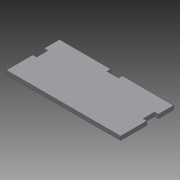
# Autodesk Inventor part: Controller_Top
Saved by Autodesk Inventor 2014 (Build 180170000, 170)
## iProperties
Created: 2014-11-10
Part Number: Controller_Top
Material: Generic
Document SubType Name: Modeling
Designer: ThatOtherGuy
Density: 1 g/cm^3
Appearance: Default
Author: ThatOtherGuy
Autodesk Inventor part; units mm, degrees
ref_plane "YZ Plane" through (0, 0, 0) normal (1, 0, 0) x (0, 1, 0)
ref_plane "XZ Plane" through (0, 0, 0) normal (0, 1, 0) x (-1, 0, 0)
ref_plane "XY Plane" through (0, 0, 0) normal (0, 0, 1) x (1, 0, 0)
sketch "Sketch1" plane through (0, 0, 0) normal (0, 0, 1) x (1, 0, 0)
  line L0 (0, 0) -> (200, 0)
  line L1 (200, 0) -> (200, 93)
  line L2 (200, 93) -> (0, 93)
  line L3 (0, 93) -> (0, 0)
  dimension "d0" = 93
  dimension "d1" = 200
  constraints: 8 end point, 2 parallel, 1 horizontal, 1 perpendicular
  measures "d0" distance of L2.end L0.start
  measures "d1" distance of L0.start L0.end
extrude "Extrusion1" add sketch "Sketch1" along normal blind 6.731
sketch "Sketch2" plane through (0, 0, 6.731) normal (0, 0, 1) x (1, 0, 0)
  line L0 (200, 0) -> (200, 93) projected
  line L1 (200, 93) -> (0, 93) projected
  line L2 (0, 93) -> (0, 0) projected
  line L3 (90, 93) -> (110, 93)
  line L4 (110, 93) -> (110, 86.269)
  line L5 (110, 86.269) -> (90, 86.269)
  line L6 (90, 86.269) -> (90, 93)
  line L7 (0, 66.269) -> (6.731, 66.269)
  line L8 (6.731, 66.269) -> (6.731, 46.269)
  line L9 (6.731, 46.269) -> (0, 46.269)
  line L10 (0, 46.269) -> (0, 66.269)
  line L11 (200, 66.269) -> (193.269, 66.269)
  line L12 (193.269, 66.269) -> (193.269, 46.269)
  line L13 (193.269, 46.269) -> (200, 46.269)
  line L14 (200, 46.269) -> (200, 66.269)
  point P0 (100, 86.269)
  point P1 (100, 93)
  dimension "d5" = 20
  dimension "d6" = 6.731
  dimension "d9" = 20
  constraints: 24 end point, 7 perpendicular, 6 parallel, 3 horizontal, 3 point on line, 2 midpoint, 1 collinear, 1 vertical alignment
  measures "d5" distance of L11.end L12.end
  measures "d6" distance of L12.end L13.end
  measures "d9" distance between parallel lines of L5 L11
extrude "Extrusion2" cut sketch "Sketch2" against normal blind 6.731
equation "\"d2\" = THICKB"
equation "\"d6\" = THICKB"
equation "\"d7\" = THICKB"
equation "\"THICKA\" = 3.175"
equation "\"THICKB\" = 6.731"
equation "\"THICKC\" = 12.7"
equation "\"THICKPLY\" = 5"
equation "\"MAGDIA\" = 9.5"
equation "\"BALLDIA\" = 12"
body "Solid1"
